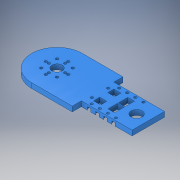
# Autodesk Inventor part: 000.401 - Опорная платформа
Saved by Autodesk Inventor 2019 (Build 230136000, 136)
## iProperties
Created: 2020-03-18
Part Number: 000.401 - Опорная платформа
Material: Пластик АБС
Document SubType Name: Modeling
Designer: Петров Иван
Density: 1.06 g/cm^3
Appearance: Голубой
Author: Петров Иван
Autodesk Inventor part; units mm, degrees
ref_plane "YZ Plane" through (0, 0, 0) normal (1, 0, 0) x (0, 1, 0)
ref_plane "XZ Plane" through (0, 0, 0) normal (0, 1, 0) x (-1, 0, 0)
ref_plane "XY Plane" through (0, 0, 0) normal (0, 0, 1) x (1, 0, 0)
sketch "Эскиз1" plane through (0, 0, 0) normal (0, 1, 0) x (-1, 0, 0)
  circle A0 centre (0, 0) radius 13.8
  circle A1 centre (-8, 0) radius 1.2
  circle A2 centre (0, -8) radius 1.2
  circle A3 centre (8, 0) radius 1.2
  circle A4 centre (0, 8) radius 1.2
  circle A5 centre (-7.7782, 7.7782) radius 1.2813
  circle A6 centre (-11, 0) radius 1.2813
  circle A7 centre (-7.7782, -7.7782) radius 1.2813
  circle A8 centre (0, -11) radius 1.2812
  circle A9 centre (7.7782, -7.7782) radius 1.2812
  circle A10 centre (11, 0) radius 1.2813
  circle A11 centre (7.7782, 7.7782) radius 1.2812
  circle A12 centre (0, 11) radius 1.2812
  circle A13 centre (0, 0) radius 5
  circle A14 centre (0, 0) radius 14
  circle A15 centre (0, 0) radius 1.55
  circle A16 centre (0, 0) radius 1.75
  circle A17 centre (0, 0) radius 25
  dimension "d0" = 50
  constraints: 18 centre point, 1 coincident
  measures "d0" diameter of A17
extrude "Выдавливание1" add sketch "Эскиз1" along normal blind 5 contours A0 | A14 | A17
sketch "Эскиз2" plane through (0, 5, 0) normal (0, 1, 0) x (1, 0, 0)
  line L0 (25, 0) -> (100, 0)
  circle A0 centre (100, 0) radius 25
  line L1 (50, 0) -> (50, -20)
  line L2 (50, 0) -> (50, 20)
  circle A1 centre (0, 0) radius 25 projected
  arc A2 (4.9455, 24.506) -> (95.0545, 24.506) centre (50, 247.5) ccw
  arc A3 (95.0545, -24.506) -> (4.9455, -24.506) centre (50, -247.5) ccw
  line L3 (100, 25) -> (0, 25)
  line L4 (0, -25) -> (100, -25)
  line L5 (50, 20) -> (50, 25)
  line L6 (50, -20) -> (50, -25)
  line L7 (50, 25) -> (50, -25)
  dimension "d3" = 100
  dimension "d4" = 50
  dimension "d5" = 20
  dimension "d6" = 20
  constraints: 16 end point, 15 point on circle, 3 centre point, 3 tangent, 2 midpoint, 2 vertical, 1 coincident, 1 collinear, 1 horizontal, 1 point on line
  measures "d3" distance of point (0, 0) L0.end
  measures "d4" diameter of A0
  measures "d5" distance of L1.start L1.end
  measures "d6" distance of L1.start L2.end
extrude "Выдавливание2" add sketch "Эскиз2" against normal blind 5 contours A1 A2 L2 L0 | L0 L1 A3 A1 | A1 L3 L5 A2 | A3 L6 L4 A1
sketch "Эскиз7" plane through (0, 5, 0) normal (0, 1, 0) x (1, 0, 0)
  line L0 (100, 0) -> (100, 15)
  line L1 (100, 0) -> (100, -15)
  circle A0 centre (100, 15) radius 3
  circle A1 centre (100, -15) radius 3
  line L2 (100, 0) -> (115, 0)
  circle A2 centre (115, 0) radius 3
  point P0 (0, 0)
  dimension "d23" = 15
  dimension "d24" = 15
  dimension "d25" = 6
  dimension "d26" = 6
  dimension "d27" = 15
  dimension "d28" = 6
  constraints: 6 end point, 3 centre point, 3 coincident, 2 vertical, 1 horizontal, 1 other
  measures "d23" distance of L0.start L0.end
  measures "d24" distance of L0.start L1.end
  measures "d25" diameter of A0
  measures "d26" diameter of A1
  measures "d27" distance of L0.start L2.end
  measures "d28" diameter of A2
extrude "Выдавливание7" [suppressed]
move faces "Перенос1" translate (40, 0, 0) faces at (50, 3.3333, 8.3333)
sketch "Эскиз10" plane through (0, 5, 0) normal (0, 1, 0) x (1, 0, 0)
  line L0 (75, -15) -> (75, -13)
  line L1 (75, -13) -> (76.5, -13)
  line L2 (76.5, -13) -> (76.5, -12)
  line L3 (76.5, -12) -> (85, -12)
  arc A0 (85, -12) -> (89, -8) centre (85, -8) ccw
  line L4 (89, -8) -> (89, 8)
  arc A1 (89, 8) -> (85, 12) centre (85, 8) ccw
  line L5 (85, 12) -> (76.5, 12)
  line L6 (76.5, 12) -> (76.5, 13)
  line L7 (76.5, 13) -> (75, 13)
  line L8 (75, 13) -> (75, 15)
  line L9 (75, 15) -> (68.5, 15)
  line L10 (68.5, 15) -> (68.5, 13)
  line L11 (68.5, 13) -> (67, 13)
  line L12 (67, 13) -> (67, 15)
  line L13 (67, 15) -> (60.5, 15)
  line L14 (60.5, 15) -> (60.5, 13)
  line L15 (60.5, 13) -> (59, 13)
  line L16 (59, 13) -> (59, 15)
  line L17 (59, 15) -> (52.5, 15)
  line L18 (52.5, 15) -> (52.5, 13)
  line L19 (52.5, 13) -> (51, 13)
  line L20 (51, 13) -> (51, 15)
  line L21 (51, 15) -> (44.5, 15)
  line L22 (44.5, 15) -> (44.5, 13)
  line L23 (44.5, 13) -> (43, 13)
  line L24 (43, 13) -> (43, 11.25)
  line L25 (43, 11.25) -> (41, 11.25)
  line L26 (41, 11.25) -> (41, 4.75)
  line L27 (41, 4.75) -> (43, 4.75)
  line L28 (43, 4.75) -> (43, -4.75)
  line L29 (43, -4.75) -> (41, -4.75)
  line L30 (41, -4.75) -> (41, -11.25)
  line L31 (41, -11.25) -> (43, -11.25)
  line L32 (43, -11.25) -> (43, -13)
  line L33 (43, -13) -> (44.5, -13)
  line L34 (44.5, -13) -> (44.5, -15)
  line L35 (44.5, -15) -> (51, -15)
  line L36 (51, -15) -> (51, -13)
  line L37 (51, -13) -> (52.5, -13)
  line L38 (52.5, -13) -> (52.5, -15)
  line L39 (52.5, -15) -> (59, -15)
  line L40 (59, -15) -> (59, -13)
  line L41 (59, -13) -> (60.5, -13)
  line L42 (60.5, -13) -> (60.5, -15)
  line L43 (60.5, -15) -> (67, -15)
  line L44 (67, -15) -> (67, -13)
  line L45 (67, -13) -> (68.5, -13)
  line L46 (68.5, -13) -> (68.5, -15)
  line L47 (68.5, -15) -> (75, -15)
  line L48 (46, -4.3) -> (46, -9.7)
  arc A2 (46.3, -4) -> (46, -4.3) centre (46.3, -4.3) ccw
  line L49 (52.7, -4) -> (46.3, -4)
  arc A3 (53, -4.3) -> (52.7, -4) centre (52.7, -4.3) ccw
  line L50 (53, -9.7) -> (53, -4.3)
  arc A4 (52.7, -10) -> (53, -9.7) centre (52.7, -9.7) ccw
  line L51 (46.3, -10) -> (52.7, -10)
  arc A5 (46, -9.7) -> (46.3, -10) centre (46.3, -9.7) ccw
  circle A6 centre (42.5, -8) radius 1.25
  circle A7 centre (47.75, -13.5) radius 1.25
  circle A8 centre (55.75, -13.5) radius 1.25
  circle A9 centre (63.75, -13.5) radius 1.25
  circle A10 centre (71.75, -13.5) radius 1.25
  circle A11 centre (42.5, 8) radius 1.25
  circle A12 centre (55.75, 13.5) radius 1.25
  circle A13 centre (71.75, 13.5) radius 1.25
  circle A14 centre (86, 6) radius 1
  circle A15 centre (72.5, -8) radius 1
  circle A16 centre (57, -8) radius 1
  circle A17 centre (86, -6) radius 1
  circle A18 centre (57, 8) radius 1
  circle A19 centre (72.5, 8) radius 1
  circle A20 centre (78.5, 0) radius 5.4
  line L52 (60, 0.5) -> (60, 9.8)
  line L53 (60, 9.8) -> (66.5, 9.8)
  line L54 (66.5, 9.8) -> (66.5, 0.5)
  line L55 (60, 0.5) -> (66.5, 0.5)
  line L56 (66.5, -0.5) -> (66.5, -9.8)
  line L57 (66.5, -9.8) -> (60, -9.8)
  line L58 (60, -9.8) -> (60, -0.5)
  line L59 (66.5, -0.5) -> (60, -0.5)
  circle A21 centre (63.75, 13.5) radius 1.25
  circle A22 centre (47.75, 13.5) radius 1.25
  line L60 (52.7, 10) -> (46.3, 10)
  arc A23 (53, 9.7) -> (52.7, 10) centre (52.7, 9.7) ccw
  line L61 (53, 4.3) -> (53, 9.7)
  arc A24 (52.7, 4) -> (53, 4.3) centre (52.7, 4.3) ccw
  line L62 (46.3, 4) -> (52.7, 4)
  arc A25 (46, 4.3) -> (46.3, 4) centre (46.3, 4.3) ccw
  line L63 (46, 9.7) -> (46, 4.3)
  arc A26 (46.3, 10) -> (46, 9.7) centre (46.3, 9.7) ccw
  line L64 (85, -13) -> (76.5, -13)
  arc A27 (85, -13) -> (90, -8) centre (85, -8) ccw
  line L65 (90, 8) -> (90, -8)
  arc A28 (90, 8) -> (85, 13) centre (85, 8) ccw
  line L66 (76.5, 13) -> (85, 13)
  line L67 (76.5, 14.5) -> (76.5, 13)
  line L68 (75, 14.5) -> (76.5, 14.5)
  line L69 (68.5, 16) -> (75, 16)
  line L70 (75, 16) -> (75, 15)
  line L71 (68.5, 15) -> (68.5, 16)
  line L72 (60.5, 16) -> (67, 16)
  line L73 (67, 16) -> (67, 15)
  line L74 (60.5, 15) -> (60.5, 16)
  line L75 (59, 16) -> (59, 15)
  line L76 (52.5, 15) -> (52.5, 16)
  line L77 (52.5, 16) -> (59, 16)
  line L78 (44.5, 16) -> (51, 16)
  line L79 (51, 16) -> (51, 15)
  line L80 (44.5, 15) -> (44.5, 16)
  line L81 (43, 14.5) -> (44.5, 14.5)
  line L82 (44.5, 14.5) -> (44.5, 13)
  line L83 (43, 14.5) -> (44.5, 14.5)
  line L84 (43, 13) -> (43, 14.5)
  line L85 (44.5, 13) -> (43, 13)
  line L86 (41.5, 13) -> (43, 13)
  line L87 (41.5, 13) -> (43, 13)
  line L88 (41.5, 11.25) -> (41.5, 13)
  line L89 (43, 11.25) -> (41.5, 11.25)
  line L90 (43, 13) -> (43, 11.25)
  line L91 (40, 4.75) -> (40, 11.25)
  line L92 (40, 11.25) -> (41, 11.25)
  line L93 (40, 4.75) -> (40, 11.25)
  line L94 (41, 4.75) -> (40, 4.75)
  line L95 (41, 11.25) -> (41, 4.75)
  line L96 (40, -4.75) -> (41, -4.75)
  line L97 (40, -11.25) -> (40, -4.75)
  line L98 (41, -11.25) -> (40, -11.25)
  line L99 (41, -4.75) -> (41, -11.25)
  line L100 (41.5, -11.25) -> (43, -11.25)
  line L101 (41.5, -13) -> (41.5, -11.25)
  line L102 (43, -13) -> (41.5, -13)
  line L103 (43, -11.25) -> (43, -13)
  line L104 (43, -14.5) -> (43, -13)
  line L105 (44.5, -14.5) -> (43, -14.5)
  line L106 (44.5, -13) -> (44.5, -14.5)
  line L107 (43, -13) -> (44.5, -13)
  line L108 (44.5, -16) -> (44.5, -15)
  line L109 (51, -16) -> (44.5, -16)
  line L110 (51, -15) -> (51, -16)
  line L111 (44.5, -15) -> (51, -15)
  line L112 (52.5, -16) -> (52.5, -15)
  line L113 (59, -16) -> (52.5, -16)
  line L114 (59, -15) -> (59, -16)
  line L115 (52.5, -15) -> (59, -15)
  line L116 (60.5, -16) -> (60.5, -15)
  line L117 (67, -16) -> (60.5, -16)
  line L118 (67, -15) -> (67, -16)
  line L119 (60.5, -15) -> (67, -15)
  line L120 (68.5, -16) -> (68.5, -15)
  line L121 (75, -16) -> (68.5, -16)
  line L122 (75, -15) -> (75, -16)
  line L123 (68.5, -15) -> (75, -15)
  line L124 (75, -14.5) -> (75, -13)
  line L125 (76.5, -14.5) -> (75, -14.5)
  line L126 (76.5, -13) -> (76.5, -14.5)
  line L127 (75, -13) -> (76.5, -13)
  line L128 (90, -25) -> (90, 25) projected
  point P0 (0, 0)
  point P1 (78.5, 0)
  point P2 (90, 0)
  point P3 (90, 0)
  constraints: 256 end point, 29 centre point, 24 point on circle, 2 midpoint
extrude "Выдавливание10" cut sketch "Эскиз10" against normal blind 10 contours A2 L49 A3 L50 A4 L51 A5 L48 | A6 | A7 | A8 | A9 | A10 | A11 | A12 | A13 | A20 | L52 L53 L54 L55 | L56 L57 L58 L59 | A21 | A22 | A23 L61 A24 L62 A25 L63 A26 L60
sketch "Эскиз11" plane through (0, 5, 0) normal (0, 1, 0) x (1, 0, 0)
  line L0 (90, -25) -> (0, -25) projected
  line L1 (90, -25) -> (40, -25)
  line L2 (40, -25) -> (40, -16)
  line L3 (40, -16) -> (90, -16)
  line L4 (90, -16) -> (90, -25)
  point P0 (0, 0)
  dimension "d41" = 50
  dimension "d42" = 9
  constraints: 8 end point, 2 parallel, 1 horizontal, 1 perpendicular
  measures "d41" distance of L2.end L3.end
  measures "d42" distance of L1.end L2.end
extrude "Выдавливание11" cut sketch "Эскиз11" against normal blind 10
mirror "Зеркальное отражение2" about plane through (0, 0, 0) normal (0, 0, 1) of "Выдавливание11"
sketch "Эскиз12" plane through (0, 0, 0) normal (0, -1, 0) x (1, 0, 0)
  circle A0 centre (47.75, 13.5) radius 1.25 projected
  circle A1 centre (47.75, 13.5) radius 3
  circle A2 centre (55.75, 13.5) radius 1.25 projected
  circle A3 centre (55.75, 13.5) radius 3
  circle A4 centre (63.75, 13.5) radius 1.25 projected
  circle A5 centre (63.75, 13.5) radius 3
  circle A6 centre (71.75, 13.5) radius 1.25 projected
  circle A7 centre (71.75, 13.5) radius 3
  circle A8 centre (42.5, 8) radius 1.25 projected
  circle A9 centre (42.5, 8) radius 3
  point P0 (0, 0)
  dimension "d46" = 6
  dimension "d47" = 6
  dimension "d48" = 6
  dimension "d49" = 6
  dimension "d50" = 6
  constraints: 5 centre point, 5 coincident
  measures "d46" diameter of A1
  measures "d47" diameter of A3
  measures "d48" diameter of A5
  measures "d49" diameter of A7
  measures "d50" diameter of A9
extrude "Выдавливание12" cut sketch "Эскиз12" against normal blind 3
mirror "Зеркальное отражение3" about plane through (0, 0, 0) normal (0, 0, 1) of "Выдавливание12"
equation "\"d6\" = d5"
equation "\"d24\" = d23"
equation "\"d26\" = d25"
equation "\"d27\" = d23"
equation "\"d28\" = d25"
equation "\"d46\" = d50"
equation "\"d47\" = d50"
equation "\"d48\" = d50"
equation "\"d49\" = d50"
